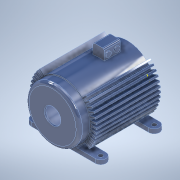
# Autodesk Inventor part: Motor_Frame_
Saved by Autodesk Inventor 2021 (Build 250183000, 183)
## iProperties
Created: 2021-07-28
Part Number: Motor_Frame_
Material: Iron, Cast
Document SubType Name: Modeling
Designer: MOGIRE
Density: 7.15 g/cm^3
Appearance: Flaked Satin - Blue
Author: MOGIRE
Autodesk Inventor part; units mm, degrees
ref_plane "YZ Plane" through (0, 0, 0) normal (1, 0, 0) x (0, 1, 0)
ref_plane "XZ Plane" through (0, 0, 0) normal (0, 1, 0) x (-1, 0, 0)
ref_plane "XY Plane" through (0, 0, 0) normal (0, 0, 1) x (1, 0, 0)
sketch "Sketch1" plane through (0, 0, 0) normal (1, 0, 0) x (0, 1, 0)
  line L0 (0, 0) -> (0, -700) construction
  line L1 (0, -700) -> (245, -700)
  line L2 (245, -700) -> (245, -115)
  line L3 (245, -115) -> (235, -115)
  line L4 (235, -115) -> (235, -30)
  line L5 (220, -15) -> (77.5, -15)
  arc A0 (235, -30) -> (220, -15) centre (220, -30) ccw
  line L6 (77.5, -15) -> (77.5, 0)
  line L7 (77.5, 0) -> (220, 0)
  line L8 (250, -30) -> (250, -100)
  line L9 (250, -100) -> (260, -100)
  line L10 (260, -100) -> (260, -700)
  line L11 (260, -700) -> (245, -700)
  arc A1 (250, -30) -> (220, 0) centre (220, -30) ccw
  point P0 (235, -15)
  point P1 (250, 0)
  dimension "d0" = 700
  dimension "d1" = 245
  dimension "d2" = 585
  dimension "d3" = 10
  dimension "d4" = 100
  dimension "d5" = 157.5
  dimension "d6" = 15
  dimension "d7" = 172.5
  dimension "d8" = 100
  dimension "d9" = 10
  dimension "d10" = 30
  constraints: 24 end point, 5 vertical, 4 horizontal, 4 point on circle, 4 point on line, 4 tangent, 2 centre point, 2 perpendicular
  measures "d0" distance of L0.start L0.end
  measures "d1" distance of L0.end L1.end
  measures "d2" distance of L1.end L2.end
  measures "d3" distance of L2.end L3.end
  measures "d4" distance of L3.end point (235, -15)
  measures "d5" distance of point (235, -15) L5.end
  measures "d6" radius of A0
  measures "d7" distance of L6.end point (250, 0)
  measures "d8" distance of point (250, 0) L8.end
  measures "d9" distance of L8.end L9.end
  measures "d10" radius of A1
revolve "Revolution1" add sketch "Sketch1" angle 360 about axis through (0, 0, 0) along (0, 0, -1)
sketch "Sketch2" plane through (0, 0, -700) normal (0, 0, -1) x (-1, 0, 0)
  circle A0 centre (0, 0) radius 245
  line L0 (350, -285) -> (-350, -285)
  line L1 (-350, -285) -> (-350, -245)
  line L2 (-350, -245) -> (350, -245)
  line L3 (350, -245) -> (350, -285)
  line L4 (350, -285) -> (-350, -245) construction
  line L5 (-350, -285) -> (350, -245) construction
  circle A1 centre (0, 0) radius 245 projected
  point P0 (0, -265)
  point P1 (0, -265)
  dimension "d12" = 40
  dimension "d13" = 490
  dimension "d14" = 700
  constraints: 12 end point, 3 midpoint, 2 parallel, 1 centre point, 1 coincident, 1 horizontal, 1 perpendicular, 1 tangent, 1 vertical alignment
  measures "d12" distance of L0.end L1.end
  measures "d13" diameter of A0
  measures "d14" distance of L0.start L0.end
extrude "Extrusion1" add sketch "Sketch2" against normal blind 100 contours L2 L3 L0 L1
fillet "Fillet1" radius 50 4 edges at (-350, -265, -700) (-350, -265, -600) (350, -265, -600) (350, -265, -700)
fillet "Fillet2" radius 10 2 edges at (87.0345, -245, -650) (-87.0345, -245, -650)
sketch "Sketch3" plane through (300, -245, -650) normal (0, 1, 0) x (1, 0, 0)
  point P0 (-300, -650)
  point P1 (0, 0)
hole "Hole1" at (300, -245, -650) direction (0, -1, 0) diameter 40 end through all
ref_plane "Work Plane1" through (300, -285, -400) normal (0, 0, -1) x (-1, 0, 0)
mirror "Mirror1" about plane through (300, -285, -400) normal (0, 0, -1) of "Fillet1", "Extrusion1", "Fillet2", "Hole1"
ref_plane "Work Plane2" through (300, -285, -580) normal (0, 0, -1) x (-1, 0, 0)
sketch "Sketch4" plane through (300, -285, -580) normal (0, 0, -1) x (-1, 0, 0)
  arc A0 (352.35, 539.6752) -> (247.65, 539.6752) centre (300, 285) ccw
  line L0 (337.35, 639.7625) -> (262.65, 639.7625)
  line L1 (247.65, 624.7625) -> (247.65, 539.6752)
  line L2 (352.35, 539.6752) -> (352.35, 624.7625)
  line L3 (352.35, 639.7625) -> (247.65, 512.7625) construction
  line L4 (247.65, 639.7625) -> (352.35, 512.7625) construction
  arc A1 (262.65, 639.7625) -> (247.65, 624.7625) centre (262.65, 624.7625) ccw
  arc A2 (352.35, 624.7625) -> (337.35, 639.7625) centre (337.35, 624.7625) ccw
  point P0 (300, 576.2625)
  dimension "d28" = 15
  constraints: 10 end point, 6 point on circle, 4 point on line, 4 tangent, 3 centre point, 2 midpoint, 1 coincident, 1 equal radius, 1 horizontal, 1 parallel, 1 perpendicular
  measures "d28" radius of A1
extrude "Extrusion2" add sketch "Sketch4" against normal blind 150
sketch "Sketch5" plane through (52.35, 254.6752, -580) normal (1, 0, 0) x (0, 0, -1)
  circle A0 centre (-34.925, 42.8625) radius 25
  circle A1 centre (-117.475, 42.8625) radius 25
  line L0 (0, 0) -> (0, 85.0873) projected
  line L1 (0, 42.5436) -> (-150, 42.5436) construction
  line L2 (-150, 85.0873) -> (-150, 0) projected
  point P0 (-580, -254.6752)
  constraints: 2 centre point, 2 end point, 2 midpoint, 1 horizontal
extrude "Extrusion3" add sketch "Sketch5" along normal blind 10
sketch "Sketch6" plane through (300, -285, -700) normal (0, 0, -1) x (-1, 0, 0)
  circle A0 centre (300, 285) radius 260
  line L0 (300, 285) -> (-9.525, 285) construction
  line L1 (40.1174, 292.8125) -> (-12.7, 292.8125)
  line L2 (-12.7, 292.8125) -> (-12.7, 277.8125)
  line L3 (-12.7, 277.8125) -> (40.0994, 277.8125)
  line L4 (38.1, 292.1875) -> (-19.05, 277.8125) construction
  line L5 (-19.05, 292.1875) -> (38.1, 277.8125) construction
  line L6 (41.321, 258.8242) -> (-11.0445, 251.9301)
  line L7 (-11.0445, 251.9301) -> (-9.0867, 237.0584)
  line L8 (-9.0867, 237.0584) -> (43.261, 243.9501)
  line L9 (46.9507, 225.2837) -> (-4.067, 211.6136)
  line L10 (-4.067, 211.6136) -> (-0.1847, 197.1247)
  line L11 (-0.1847, 197.1247) -> (50.8155, 210.7902)
  line L12 (56.9101, 192.765) -> (8.1132, 172.5527)
  line L13 (8.1132, 172.5527) -> (13.8534, 158.6945)
  line L14 (13.8534, 158.6945) -> (62.6337, 178.8999)
  line L15 (71.0288, 161.8245) -> (25.2876, 135.4158)
  line L16 (25.2876, 135.4158) -> (32.7876, 122.4254)
  line L17 (32.7876, 122.4254) -> (78.5132, 148.8251)
  line L18 (89.0653, 132.9916) -> (47.1625, 100.8384)
  line L19 (47.1625, 100.8384) -> (56.2939, 88.9381)
  line L20 (56.2939, 88.9381) -> (98.1824, 121.0803)
  line L21 (110.711, 106.7595) -> (73.3634, 69.412)
  line L22 (73.3634, 69.412) -> (83.97, 58.8054)
  line L23 (83.97, 58.8054) -> (121.3048, 96.1402)
  line L24 (135.5954, 83.5772) -> (103.4422, 41.6744)
  line L25 (103.4422, 41.6744) -> (115.3425, 32.5429)
  line L26 (115.3425, 32.5429) -> (147.4847, 74.4315)
  line L27 (163.2929, 63.8413) -> (136.8842, 18.1001)
  line L28 (136.8842, 18.1001) -> (149.8746, 10.6001)
  line L29 (149.8746, 10.6001) -> (176.2742, 56.3257)
  line L30 (193.3294, 47.8895) -> (173.1171, -0.9074)
  line L31 (173.1171, -0.9074) -> (186.9753, -6.6477)
  line L32 (186.9753, -6.6477) -> (207.1807, 42.1326)
  line L33 (225.1911, 35.9947) -> (211.521, -15.023)
  line L34 (211.521, -15.023) -> (226.0099, -18.9053)
  line L35 (226.0099, -18.9053) -> (239.6754, 32.095)
  line L36 (258.3329, 28.3605) -> (251.4388, -24.0051)
  line L37 (251.4388, -24.0051) -> (266.3105, -25.963)
  line L38 (266.3105, -25.963) -> (273.2022, 26.3847)
  line L39 (292.1875, 25.1174) -> (292.1875, -27.7)
  line L40 (292.1875, -27.7) -> (307.1875, -27.7)
  line L41 (307.1875, -27.7) -> (307.1875, 25.0994)
  line L42 (326.1758, 26.321) -> (333.0699, -26.0445)
  line L43 (333.0699, -26.0445) -> (347.9416, -24.0867)
  line L44 (347.9416, -24.0867) -> (341.0499, 28.261)
  line L45 (359.7163, 31.9507) -> (373.3864, -19.067)
  line L46 (373.3864, -19.067) -> (387.8753, -15.1847)
  line L47 (387.8753, -15.1847) -> (374.2098, 35.8155)
  line L48 (392.235, 41.9101) -> (412.4473, -6.8868)
  line L49 (412.4473, -6.8868) -> (426.3055, -1.1466)
  line L50 (426.3055, -1.1466) -> (406.1001, 47.6337)
  line L51 (423.1755, 56.0288) -> (449.5842, 10.2876)
  line L52 (449.5842, 10.2876) -> (462.5746, 17.7876)
  line L53 (462.5746, 17.7876) -> (436.1749, 63.5132)
  line L54 (452.0084, 74.0653) -> (484.1616, 32.1625)
  line L55 (484.1616, 32.1625) -> (496.0619, 41.2939)
  line L56 (496.0619, 41.2939) -> (463.9197, 83.1824)
  line L57 (478.2405, 95.711) -> (515.588, 58.3634)
  line L58 (515.588, 58.3634) -> (526.1946, 68.97)
  line L59 (526.1946, 68.97) -> (488.8598, 106.3048)
  line L60 (501.4228, 120.5954) -> (543.3256, 88.4422)
  line L61 (543.3256, 88.4422) -> (552.4571, 100.3425)
  line L62 (552.4571, 100.3425) -> (510.5685, 132.4847)
  line L63 (521.1587, 148.2929) -> (566.8999, 121.8842)
  line L64 (566.8999, 121.8842) -> (574.3999, 134.8746)
  line L65 (574.3999, 134.8746) -> (528.6743, 161.2742)
  line L66 (537.1105, 178.3294) -> (585.9074, 158.1171)
  line L67 (585.9074, 158.1171) -> (591.6477, 171.9753)
  line L68 (591.6477, 171.9753) -> (542.8674, 192.1807)
  line L69 (549.0053, 210.1911) -> (600.023, 196.521)
  line L70 (600.023, 196.521) -> (603.9053, 211.0099)
  line L71 (603.9053, 211.0099) -> (552.905, 224.6754)
  line L72 (556.6395, 243.3329) -> (609.0051, 236.4388)
  line L73 (609.0051, 236.4388) -> (610.963, 251.3105)
  line L74 (610.963, 251.3105) -> (558.6153, 258.2022)
  line L75 (559.8826, 277.1875) -> (612.7, 277.1875)
  line L76 (612.7, 277.1875) -> (612.7, 292.1875)
  line L77 (612.7, 292.1875) -> (559.9006, 292.1875)
  line L78 (558.679, 311.1758) -> (611.0445, 318.0699)
  line L79 (611.0445, 318.0699) -> (609.0867, 332.9416)
  line L80 (609.0867, 332.9416) -> (556.739, 326.0499)
  line L81 (553.0493, 344.7163) -> (604.067, 358.3864)
  line L82 (604.067, 358.3864) -> (600.1847, 372.8753)
  line L83 (600.1847, 372.8753) -> (549.1845, 359.2098)
  line L84 (543.0899, 377.235) -> (591.8868, 397.4473)
  line L85 (591.8868, 397.4473) -> (586.1466, 411.3055)
  line L86 (586.1466, 411.3055) -> (537.3663, 391.1001)
  line L87 (528.9712, 408.1755) -> (574.7124, 434.5842)
  line L88 (574.7124, 434.5842) -> (567.2124, 447.5746)
  line L89 (567.2124, 447.5746) -> (521.4868, 421.1749)
  line L90 (510.9347, 437.0084) -> (552.8375, 469.1616)
  line L91 (552.8375, 469.1616) -> (543.7061, 481.0619)
  line L92 (543.7061, 481.0619) -> (501.8176, 448.9197)
  line L93 (489.289, 463.2405) -> (526.6366, 500.588)
  line L94 (526.6366, 500.588) -> (516.03, 511.1946)
  line L95 (516.03, 511.1946) -> (478.6952, 473.8598)
  line L96 (464.4046, 486.4228) -> (496.5578, 528.3256)
  line L97 (496.5578, 528.3256) -> (484.6575, 537.4571)
  line L98 (484.6575, 537.4571) -> (452.5153, 495.5685)
  line L99 (436.7071, 506.1587) -> (463.1158, 551.8999)
  line L100 (463.1158, 551.8999) -> (450.1254, 559.3999)
  line L101 (450.1254, 559.3999) -> (423.7258, 513.6743)
  line L102 (406.6706, 522.1105) -> (426.8829, 570.9074)
  line L103 (426.8829, 570.9074) -> (413.0247, 576.6477)
  line L104 (413.0247, 576.6477) -> (392.8193, 527.8674)
  line L105 (374.8089, 534.0053) -> (388.479, 585.023)
  line L106 (388.479, 585.023) -> (373.9901, 588.9053)
  line L107 (373.9901, 588.9053) -> (360.3246, 537.905)
  line L108 (341.6671, 541.6395) -> (348.5612, 594.0051)
  line L109 (348.5612, 594.0051) -> (333.6895, 595.963)
  line L110 (333.6895, 595.963) -> (326.7978, 543.6153)
  line L111 (307.8125, 544.8826) -> (307.8125, 597.7)
  line L112 (307.8125, 597.7) -> (292.8125, 597.7)
  line L113 (292.8125, 597.7) -> (292.8125, 544.9006)
  line L114 (273.8242, 543.679) -> (266.9301, 596.0445)
  line L115 (266.9301, 596.0445) -> (252.0584, 594.0867)
  line L116 (252.0584, 594.0867) -> (258.9501, 541.739)
  line L117 (240.2837, 538.0493) -> (226.6136, 589.067)
  line L118 (226.6136, 589.067) -> (212.1247, 585.1847)
  line L119 (212.1247, 585.1847) -> (225.7902, 534.1845)
  line L120 (207.765, 528.0899) -> (187.5527, 576.8868)
  line L121 (187.5527, 576.8868) -> (173.6945, 571.1466)
  line L122 (173.6945, 571.1466) -> (193.8999, 522.3663)
  line L123 (176.8245, 513.9712) -> (150.4158, 559.7124)
  line L124 (150.4158, 559.7124) -> (137.4254, 552.2124)
  line L125 (137.4254, 552.2124) -> (163.8251, 506.4868)
  line L126 (147.9916, 495.9347) -> (115.8384, 537.8375)
  line L127 (115.8384, 537.8375) -> (103.9381, 528.7061)
  line L128 (103.9381, 528.7061) -> (136.0803, 486.8176)
  line L129 (121.7595, 474.289) -> (84.412, 511.6366)
  line L130 (84.412, 511.6366) -> (73.8054, 501.03)
  line L131 (73.8054, 501.03) -> (111.1402, 463.6952)
  line L132 (98.5772, 449.4046) -> (56.6744, 481.5578)
  line L133 (56.6744, 481.5578) -> (47.5429, 469.6575)
  line L134 (47.5429, 469.6575) -> (89.4315, 437.5153)
  line L135 (78.8413, 421.7071) -> (33.1001, 448.1158)
  line L136 (33.1001, 448.1158) -> (25.6001, 435.1254)
  line L137 (25.6001, 435.1254) -> (71.3257, 408.7258)
  line L138 (62.8895, 391.6706) -> (14.0926, 411.8829)
  line L139 (14.0926, 411.8829) -> (8.3523, 398.0247)
  line L140 (8.3523, 398.0247) -> (57.1326, 377.8193)
  line L141 (50.9947, 359.8089) -> (-0.023, 373.479)
  line L142 (-0.023, 373.479) -> (-3.9053, 358.9901)
  line L143 (-3.9053, 358.9901) -> (47.095, 345.3246)
  line L144 (43.3605, 326.6671) -> (-9.0051, 333.5612)
  line L145 (-9.0051, 333.5612) -> (-10.963, 318.6895)
  line L146 (-10.963, 318.6895) -> (41.3847, 311.7978)
  point P0 (9.525, 285)
  point P1 (537.3663, 391.1001)
  point P2 (549.0053, 210.1911)
  point P3 (510.5685, 132.4847)
  point P4 (501.4228, 120.5954)
  point P5 (98.1824, 121.0803)
  point P6 (89.0653, 132.9916)
  point P7 (78.5132, 148.8251)
  point P8 (71.0288, 161.8245)
  point P9 (56.9101, 192.765)
  point P10 (46.9507, 225.2837)
  point P11 (41.3847, 311.7978)
  point P12 (43.3605, 326.6671)
  point P13 (47.095, 345.3246)
  point P14 (57.1326, 377.8193)
  point P15 (89.4315, 437.5153)
  point P16 (98.5772, 449.4046)
  dimension "d35" = 15
  dimension "d38" = 360
  constraints: 294 end point, 2 horizontal, 2 midpoint, 1 coincident, 1 parallel, 1 perpendicular, 1 point on line, 341 other
  measures "d35" distance of L1.end L2.end
extrude "Extrusion4" add sketch "Sketch6" against normal blind 600 contours A0 L77 L76 L75 | A0 L80 L79 L78 | L74 L73 L72 A0 | A0 L83 L82 L81 | L71 L70 L69 A0 | A0 L86 L85 L84 | L68 L67 L66 A0 | A0 L89 L88 L87 | L65 L64 L63 A0 | A0 L92 L91 L90 | L62 L61 L60 A0 | A0 L95 L94 L93 | A0 L131 L130 L129 | A0 L134 L133 L132 | L20 L19 L18 A0 | A0 L137 L136 L135 | L17 L16 L15 A0 | A0 L140 L139 L138 | L14 L13 L12 A0 | A0 L143 L142 L141 | L11 L10 L9 A0 | A0 L146 L145 L144 | L8 L7 L6 A0 | A0 L3 L2 L1
ref_plane "Work Plane3" through (300, -285, -615) normal (0, 0, -1) x (-1, 0, 0)
sketch "Sketch7" plane through (300, -285, -615) normal (0, 0, -1) x (-1, 0, 0)
  line L0 (25.6001, 435.1254) -> (33.1001, 448.1158) projected
  line L1 (57.1326, 377.8193) -> (8.3523, 398.0247) projected
  point P0 (300, 285)
body "Solid1"
